Autodesk Fusion 360 part; units mm, degrees
(part 2 of 2)
sketch "Sketch1" plane through (0, 0, 0) normal (1, 0, 0) x (0, 1, 0)
  line L0 (25.4, 0) -> (25.4, -3.175)
  line L1 (12.7, 0) -> (12.7, -3.175)
  line L2 (76.2, 25.4) -> (76.2, 12.7)
  line L3 (0, 0) -> (0, 25.4)
  line L4 (0, 12.7) -> (-3.175, 12.7)
  line L5 (76.2, 12.7) -> (79.375, 12.7)
  line L6 (-3.175, 25.4) -> (0, 25.4)
  line L7 (63.5, -3.175) -> (63.5, 0)
  line L8 (50.8, 0) -> (50.8, -3.175)
  line L9 (79.375, 12.7) -> (79.375, 25.4)
  line L10 (0, -3.175) -> (0, 0)
  line L11 (0, 0) -> (0, 12.7)
  line L12 (25.4, -3.175) -> (38.1, -3.175)
  line L13 (-3.175, 12.7) -> (-3.175, 25.4)
  line L14 (79.375, 25.4) -> (76.2, 25.4)
  line L15 (0, 0) -> (-7.62, 0)
  line L16 (0, 0) -> (-5.715, 0)
  line L17 (-5.715, 0) -> (-5.715, 38.1)
  line L18 (-5.715, 38.1) -> (-5.715, 43.815)
  line L19 (-5.715, 43.815) -> (76.2, 43.815)
  line L20 (76.2, 43.815) -> (81.915, 43.815)
  line L21 (81.915, 43.815) -> (81.915, 0)
  line L22 (81.915, 0) -> (81.915, -5.715)
  line L23 (81.915, -5.715) -> (0, -5.715)
  line L24 (0, -5.715) -> (-5.715, -5.715)
  line L25 (-5.715, -5.715) -> (-5.715, 0)
  line L26 (-5.715, 43.815) -> (12.7, 43.815)
  line L27 (12.7, 43.815) -> (12.7, 40.64)
  line L28 (12.7, 40.64) -> (12.7, 27.94)
  line L29 (81.915, 43.815) -> (63.5, 43.815)
  line L30 (63.5, 43.815) -> (63.5, 27.94)
  line L31 (63.5, 27.94) -> (12.7, 27.94)
  line L32 (12.7, 40.64) -> (63.5, 40.64)
  line L33 (63.5, -3.175) -> (50.8, -3.175)
  line L34 (63.5, 0) -> (50.8, 0)
  line L35 (25.4, -3.175) -> (12.7, -3.175)
  line L36 (12.7, 0) -> (25.4, 0)
  dimension "d2" = 12.7
  dimension "d3" = 3.175
  dimension "d4" = 12.7
  dimension "d6" = 12.7
  dimension "d9" = 12.7
  dimension "d10" = 3.175
  dimension "d12" = 12.7
  dimension "d13" = 3.175
  dimension "d14" = 12.7
  dimension "d16" = 3.175
  dimension "d17" = 12.7
  dimension "d18" = 7.62
  dimension "d21" = 5.715
  dimension "d22" = 5.715
  dimension "d23" = 5.715
  dimension "d24" = 5.715
  dimension "d25" = 3.175
  dimension "d26" = 12.7
  dimension "d27" = 18.415
  constraint coincident L3.start L10.end
  constraint perpendicular L0 L12
  constraint perpendicular L3 L4
  constraint perpendicular L4 L13
  constraint perpendicular L3 L6
  constraint perpendicular L2 L5
  constraint perpendicular L5 L9
  constraint perpendicular L2 L14
  constraint perpendicular L3 L15
  constraint perpendicular L3 L16
  constraint perpendicular L15 L17
  constraint perpendicular L15 L18
  constraint perpendicular L18 L19
  constraint perpendicular L18 L20
  constraint perpendicular L20 L21
  constraint perpendicular L20 L22
  constraint perpendicular L22 L23
  constraint perpendicular L22 L24
  constraint perpendicular L15 L25
  constraint coincident L19 L26.end
  constraint perpendicular L18 L26
  constraint perpendicular L26 L27
  constraint parallel L27 L28
  constraint perpendicular L21 L29
  constraint perpendicular L19 L30
  constraint coincident L30 L32.end
  constraint perpendicular L30 L32
  constraint perpendicular L8 L33
  constraint perpendicular L8 L34
  constraint perpendicular L1 L35
  constraint perpendicular L0 L36
  measures "d2" distance of L1.start L3.start
  measures "d3" distance of L1.start L1.end
  measures "d4" distance of L1.start L0.start
  measures "d6" distance of L0.end L12.end
  measures "d9" distance of L7.end L8.start
  measures "d10" distance of L8.start L8.end
  measures "d12" distance of L3.start L4.start
  measures "d13" distance of L4.end L4.start
  measures "d14" distance of L6.start L4.end
  measures "d16" distance of L5.end L2.end
  measures "d17" distance of L5.end L9.end
  measures "d18" distance of L3.start L15.end
  measures "d21" distance of L3.start L16.end
  measures "d22" distance of L17.end L18.end
  measures "d23" distance of L19.end L20.end
  measures "d24" distance of L21.end L22.end
  measures "d25" distance of L26.end L27.end
  measures "d26" distance of L27.end L28.end
  measures "d27" distance of L20.end L29.end
extrude "Extrude1" add sketch "Sketch1" along normal blind 3.175 contours L17 L18 L19 L20 L21 L22 L23 L24 L25 L26 L27 L28 L29 L30 L31 | L19 L27 L30 L32

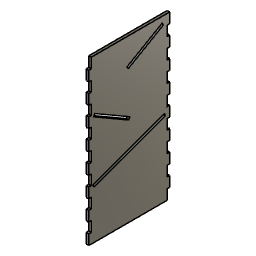
design "Dice Tower (Right Side)"
Autodesk Fusion 360 part; units mm, degrees
sketch "Sketch1" plane through (0, 0, 0) normal (1, 0, 0) x (0, 1, 0)
  line L0 (98.425, 139.7) -> (101.6, 139.7)
  line L1 (0, 101.6) -> (0, 114.3)
  line L2 (0, 127) -> (0, 139.7)
  line L3 (98.425, 114.3) -> (101.6, 114.3)
  line L4 (0, 127) -> (3.175, 127)
  line L5 (101.6, 101.6) -> (101.6, 88.9)
  line L6 (0, 101.6) -> (3.175, 101.6)
  line L7 (98.425, 0) -> (98.425, 203.2)
  line L8 (98.425, 114.3) -> (98.425, 101.6)
  line L9 (98.425, 88.9) -> (101.6, 88.9)
  line L10 (101.6, 0) -> (100.0125, 0)
  line L11 (98.425, 127) -> (101.6, 127)
  line L12 (98.425, 101.6) -> (101.6, 101.6)
  line L13 (98.425, 95.25) -> (98.425, 88.9)
  line L14 (3.175, 0) -> (3.175, 203.2)
  line L15 (101.6, 127) -> (101.6, 114.3)
  line L16 (3.175, 127) -> (3.175, 114.3)
  line L17 (3.175, 88.9) -> (0, 88.9)
  line L18 (98.425, 139.7) -> (98.425, 127)
  line L19 (3.175, 114.3) -> (0, 114.3)
  line L20 (3.175, 12.7) -> (3.175, 0)
  line L21 (3.175, 190.5) -> (3.175, 177.8)
  line L22 (3.175, 177.8) -> (0, 177.8)
  line L23 (101.6, 50.8) -> (101.6, 38.1)
  line L24 (3.175, 50.8) -> (3.175, 38.1)
  line L25 (98.425, 152.4) -> (101.6, 152.4)
  line L26 (98.425, 50.8) -> (101.6, 50.8)
  line L27 (98.425, 152.4) -> (98.425, 139.7)
  line L28 (3.175, 139.7) -> (0, 139.7)
  line L29 (0, 139.7) -> (0, 127)
  line L30 (3.175, 101.6) -> (3.175, 88.9)
  line L31 (98.425, 101.6) -> (98.425, 95.25)
  line L32 (98.425, 203.2) -> (98.425, 190.5)
  line L33 (101.6, 152.4) -> (101.6, 139.7)
  line L34 (101.6, 203.2) -> (101.6, 190.5)
  line L35 (3.175, 203.2) -> (3.175, 190.5)
  line L36 (0, 0) -> (11.0998, 0)
  line L37 (98.425, 177.8) -> (98.425, 165.1)
  line L38 (98.425, 127) -> (98.425, 114.3)
  line L39 (0, 165.1) -> (0, 152.4)
  line L40 (11.0998, 0) -> (6.0198, 0)
  line L41 (98.425, 88.9) -> (98.425, 76.2)
  line L42 (0, 38.1) -> (3.175, 38.1)
  line L43 (98.425, 38.1) -> (98.425, 25.4)
  line L44 (101.6, 177.8) -> (101.6, 165.1)
  line L45 (98.425, 12.7) -> (101.6, 12.7)
  line L46 (0, 177.8) -> (0, 190.5)
  line L47 (98.425, 177.8) -> (101.6, 177.8)
  line L48 (0, 76.2) -> (0, 88.9)
  line L49 (0, 114.3) -> (0, 101.6)
  line L50 (3.175, 190.5) -> (0, 190.5)
  line L51 (98.425, 190.5) -> (101.6, 190.5)
  line L52 (101.6, 0) -> (0, 0)
  line L53 (98.425, 38.1) -> (101.6, 38.1)
  line L54 (90.5002, 0) -> (95.5802, 0)
  line L55 (3.175, 203.2) -> (101.6, 203.2)
  line L56 (98.425, 76.2) -> (101.6, 76.2)
  line L57 (98.425, 165.1) -> (101.6, 165.1)
  line L58 (98.425, 63.5) -> (98.425, 50.8)
  line L59 (98.425, 25.4) -> (101.6, 25.4)
  line L60 (0, 0) -> (0, 12.7)
  line L61 (3.175, 63.5) -> (0, 63.5)
  line L62 (98.425, 63.5) -> (101.6, 63.5)
  line L63 (0, 152.4) -> (0, 165.1)
  line L64 (0, 152.4) -> (3.175, 152.4)
  line L65 (0, 25.4) -> (0, 38.1)
  line L66 (0, 0) -> (12.065, 0)
  line L67 (3.175, 50.8) -> (0, 50.8)
  line L68 (101.6, 203.2) -> (98.425, 203.2)
  line L69 (98.425, 190.5) -> (98.425, 177.8)
  line L70 (101.6, 76.2) -> (101.6, 63.5)
  line L71 (101.6, 0) -> (90.5002, 0)
  line L72 (3.175, 25.4) -> (3.175, 12.7)
  line L73 (98.425, 25.4) -> (98.425, 12.7)
  line L74 (3.175, 38.1) -> (3.175, 25.4)
  line L75 (0, 12.7) -> (3.175, 12.7)
  line L76 (0, 50.8) -> (0, 63.5)
  line L77 (0, 25.4) -> (3.175, 25.4)
  line L78 (3.175, 177.8) -> (3.175, 165.1)
  line L79 (101.6, 0) -> (98.425, 0)
  line L80 (101.6, 0) -> (85.725, 0)
  line L81 (101.6, 25.4) -> (101.6, 12.7)
  line L82 (3.175, 76.2) -> (0, 76.2)
  line L83 (98.425, 165.1) -> (98.425, 152.4)
  line L84 (3.175, 63.5) -> (3.175, 50.8)
  line L85 (3.175, 152.4) -> (3.175, 139.7)
  line L86 (98.425, 76.2) -> (98.425, 63.5)
  line L87 (3.175, 165.1) -> (0, 165.1)
  line L88 (98.425, 50.8) -> (98.425, 38.1)
  line L89 (3.175, 76.2) -> (3.175, 63.5)
  line L90 (0, 0) -> (3.175, 0)
  line L91 (3.175, 88.9) -> (3.175, 76.2)
  line L92 (98.425, 203.2) -> (98.425, 177.8)
  line L93 (3.175, 0) -> (3.175, 59.055)
  line L94 (7.62, 139.7) -> (51.5837, 114.2474)
  line L95 (49.9801, 111.4777) -> (6.0165, 136.9303)
  line L96 (6.0165, 136.9303) -> (7.62, 139.7)
  line L97 (93.7411, 193.04) -> (49.7434, 167.6463)
  line L98 (92.1413, 195.8119) -> (93.7411, 193.04)
  line L99 (48.1436, 170.4182) -> (92.1413, 195.8119)
  line L100 (3.175, 60.2676) -> (4.1957, 60.2676)
  line L101 (4.1957, 60.2676) -> (6.35, 60.2676)
  line L102 (6.35, 60.2676) -> (95.8689, 92.8088)
  line L103 (94.7755, 95.8167) -> (5.2566, 63.2754)
  line L104 (49.9801, 111.4777) -> (50.2, 111.3504)
  line L105 (50.2, 111.3504) -> (51.8035, 114.1201)
  line L106 (51.8035, 114.1201) -> (51.5837, 114.2474)
  line L107 (95.8689, 92.8088) -> (96.1076, 92.8956)
  line L108 (96.1076, 92.8956) -> (95.0142, 95.9034)
  line L109 (95.0142, 95.9034) -> (94.7755, 95.8167)
  line L110 (49.7434, 167.6463) -> (49.5234, 167.5194)
  line L111 (49.5234, 167.5194) -> (47.9236, 170.2912)
  line L112 (47.9236, 170.2912) -> (48.1436, 170.4182)
  line L113 (5.2566, 63.2754) -> (6.35, 60.2676)
  dimension "d9" = 11.0998
  dimension "d10" = 11.0998
  dimension "d14" = 5.08
  dimension "d15" = 5.08
  dimension "d27" = 3.175
  dimension "d28" = 3.175
  dimension "d40" = 3.175
  dimension "d41" = 3.175
  dimension "d42" = 12.7
  dimension "d43" = 12.7
  dimension "d44" = 12.7
  dimension "d45" = 12.7
  dimension "d46" = 12.7
  dimension "d47" = 12.7
  dimension "d48" = 12.7
  dimension "d49" = 12.7
  dimension "d50" = 6.35
  dimension "d51" = 6.35
  dimension "d52" = 12.7
  dimension "d53" = 12.7
  dimension "d54" = 12.7
  dimension "d55" = 12.7
  dimension "d56" = 12.7
  dimension "d57" = 12.7
  dimension "d74" = 59.055
  dimension "d78" = 50.8
  dimension "d79" = 3.2004
  dimension "d80" = 50.8
  dimension "d81" = 50.8
  dimension "d82" = 3.2004
  dimension "d83" = 50.8
  dimension "d84" = 95.25
  dimension "d85" = 3.2004
  dimension "d86" = 95.25
  dimension "d87" = 0.254
  dimension "d88" = 0.254
  dimension "d89" = 3.2004
  dimension "d90" = 0.254
  dimension "d91" = 3.2004
  constraint coincident L36.start L52.end
  constraint vertical L60
  constraint perpendicular L55 L60
  constraint perpendicular L34 L55
  constraint perpendicular L52 L60
  constraint perpendicular L60 L66
  constraint perpendicular L34 L80
  constraint perpendicular L10 L34
  constraint coincident L54.start L52
  constraint perpendicular L36 L60
  constraint perpendicular L50 L60
  constraint perpendicular L21 L50
  constraint coincident L22.end L60
  constraint perpendicular L22 L60
  constraint perpendicular L22 L78
  constraint perpendicular L60 L87
  constraint collinear L46 L60
  constraint perpendicular L39 L87
  constraint perpendicular L39 L64
  constraint parallel L66 L90
  constraint perpendicular L14 L55
  constraint perpendicular L64 L85
  constraint perpendicular L28 L60
  constraint perpendicular L28 L29
  constraint coincident L4.end L14
  constraint perpendicular L4 L14
  constraint perpendicular L4 L16
  constraint perpendicular L16 L19
  constraint perpendicular L19 L49
  constraint midpoint L6.end L14
  constraint perpendicular L6 L14
  constraint perpendicular L6 L30
  constraint parallel L14 L91
  constraint parallel L14 L89
  constraint parallel L14 L84
  constraint parallel L14 L24
  constraint parallel L24 L74
  constraint parallel L14 L72
  constraint perpendicular L17 L60
  constraint coincident L48.start L60
  constraint perpendicular L60 L82
  constraint perpendicular L60 L61
  constraint coincident L67.end L60
  constraint perpendicular L60 L67
  constraint coincident L65.start L60
  constraint collinear L60 L63
  constraint collinear L2 L60
  constraint collinear L1 L60
  constraint collinear L48 L60
  constraint collinear L60 L76
  constraint collinear L60 L65
  constraint perpendicular L34 L68
  constraint perpendicular L34 L79
  constraint perpendicular L32 L55
  constraint perpendicular L34 L51
  constraint perpendicular L51 L69
  constraint coincident L44.start L34
  constraint perpendicular L34 L47
  constraint perpendicular L37 L47
  constraint coincident L44.end L34
  constraint perpendicular L34 L57
  constraint perpendicular L57 L83
  constraint coincident L25.end L34
  constraint perpendicular L25 L34
  constraint perpendicular L25 L27
  constraint coincident L0.end L34
  constraint perpendicular L0 L34
  constraint perpendicular L0 L18
  constraint coincident L11.end L34
  constraint perpendicular L11 L34
  constraint perpendicular L11 L38
  constraint coincident L3.end L34
  constraint perpendicular L3 L34
  constraint perpendicular L3 L8
  constraint perpendicular L12 L34
  constraint perpendicular L12 L31
  constraint parallel L7 L13
  constraint coincident L5.end L34
  constraint perpendicular L9 L34
  constraint perpendicular L9 L41
  constraint coincident L56.end L34
  constraint perpendicular L34 L56
  constraint perpendicular L56 L86
  constraint coincident L62.end L34
  constraint perpendicular L34 L62
  constraint perpendicular L58 L62
  constraint coincident L23.start L34
  constraint perpendicular L26 L34
  constraint perpendicular L26 L88
  constraint coincident L23.end L34
  constraint perpendicular L34 L53
  constraint perpendicular L43 L53
  constraint perpendicular L43 L59
  constraint perpendicular L59 L73
  constraint perpendicular L45 L73
  constraint collinear L34 L44
  constraint coincident L5.start L34
  constraint collinear L33 L44
  constraint collinear L15 L33
  constraint collinear L5 L15
  constraint collinear L5 L70
  constraint collinear L23 L70
  constraint collinear L23 L81
  constraint coincident L84 L93.end
  constraint coincident L84 L100.start
  constraint perpendicular L84 L100
  constraint perpendicular L93 L101
  constraint perpendicular L95 L105
  constraint parallel L102 L107
  constraint perpendicular L107 L108
  constraint parallel L97 L110
  constraint perpendicular L110 L111
  constraint perpendicular L111 L112
  constraint perpendicular L102 L113
  measures "d9" distance of L10.start L54.start
  measures "d10" distance of L36.start L36.end
  measures "d14" distance of L36.end L40.end
  measures "d15" distance of L54.end L54.start
  measures "d27" distance of L39.end L64.end
  measures "d28" distance of L36.start L14.start
  measures "d40" distance of L7.end L34.start
  measures "d41" distance of L7.start L10.start
  measures "d42" distance of L7.end L32.end
  measures "d43" distance of L32.end L37.start
  measures "d44" distance of L37.end L37.start
  measures "d45" distance of L25.start L37.end
  measures "d46" distance of L0.start L25.start
  measures "d47" distance of L0.start L11.start
  measures "d48" distance of L3.start L11.start
  measures "d49" distance of L8.end L3.start
  measures "d50" distance of L8.end L13.start
  measures "d51" distance of L13.start L9.start
  measures "d52" distance of L9.start L41.end
  measures "d53" distance of L41.end L58.start
  measures "d54" distance of L58.start L26.start
  measures "d55" distance of L26.start L43.start
  measures "d56" distance of L43.end L43.start
  measures "d57" distance of L43.end L45.start
  measures "d74" distance of L14.start L93.end
  measures "d78" distance of L94.start L94.end
  measures "d79" distance of L95.start L94.end
  measures "d80" distance of L95.start L95.end
  measures "d81" distance of L97.start L97.end
  measures "d82" distance of L99.start L97.end
  measures "d83" distance of L98.start L99.start
  measures "d84" distance of L101.end L102.end
  measures "d85" distance of L102.end L103.start
  measures "d86" distance of L103.start L103.end
  measures "d87" distance of L95.start L104.end
  measures "d88" distance of L102.end L107.end
  measures "d89" distance of L107.end L108.end
  measures "d90" distance of L97.end L110.end
  measures "d91" distance of L110.end L111.end
extrude "Extrude1" add sketch "Sketch1" along normal blind 3.175
sketch "Sketch2" plane through (0, 0, 0) normal (1, 0, 0) x (0, 1, 0)
equation "d9 = 0.5 in - 0.063 in"

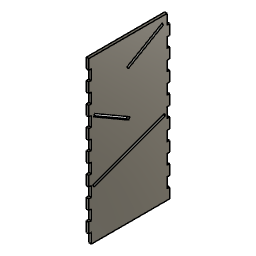
design "Dice Tower (Left Side)"
Autodesk Fusion 360 part; units mm, degrees
sketch "Sketch1" plane through (0, 0, 0) normal (1, 0, 0) x (0, 1, 0)
  line L0 (-98.425, 88.9) -> (-101.6, 88.9)
  line L1 (-98.425, 38.1) -> (-98.425, 25.4)
  line L2 (-98.425, 76.2) -> (-101.6, 76.2)
  line L3 (-101.6, 0) -> (-100.0125, 0)
  line L4 (-98.425, 190.5) -> (-98.425, 177.8)
  line L5 (-101.6, 203.2) -> (-98.425, 203.2)
  line L6 (-98.425, 177.8) -> (-98.425, 165.1)
  line L7 (-98.425, 203.2) -> (-98.425, 177.8)
  line L8 (-3.175, 177.8) -> (0, 177.8)
  line L9 (-98.425, 127) -> (-101.6, 127)
  line L10 (-3.175, 165.1) -> (0, 165.1)
  line L11 (-98.425, 165.1) -> (-98.425, 152.4)
  line L12 (0, 12.7) -> (-3.175, 12.7)
  line L13 (0, 127) -> (-3.175, 127)
  line L14 (-101.6, 76.2) -> (-101.6, 63.5)
  line L15 (-98.425, 63.5) -> (-98.425, 50.8)
  line L16 (-98.425, 114.3) -> (-98.425, 101.6)
  line L17 (-101.6, 101.6) -> (-101.6, 88.9)
  line L18 (-101.6, 0) -> (-98.425, 0)
  line L19 (-98.425, 63.5) -> (-101.6, 63.5)
  line L20 (-101.6, 0) -> (-90.5002, 0)
  line L21 (-3.175, 190.5) -> (-3.175, 177.8)
  line L22 (-3.175, 50.8) -> (0, 50.8)
  line L23 (0, 25.4) -> (-3.175, 25.4)
  line L24 (-3.175, 152.4) -> (-3.175, 139.7)
  line L25 (0, 38.1) -> (-3.175, 38.1)
  line L26 (-101.6, 177.8) -> (-101.6, 165.1)
  line L27 (0, 0) -> (-3.175, 0)
  line L28 (-3.175, 190.5) -> (0, 190.5)
  line L29 (-3.175, 50.8) -> (-3.175, 38.1)
  line L30 (-101.6, 203.2) -> (-101.6, 190.5)
  line L31 (-101.6, 127) -> (-101.6, 114.3)
  line L32 (-98.425, 114.3) -> (-101.6, 114.3)
  line L33 (0, 0) -> (-11.0998, 0)
  line L34 (-98.425, 139.7) -> (-98.425, 127)
  line L35 (-3.175, 177.8) -> (-3.175, 165.1)
  line L36 (-98.425, 165.1) -> (-101.6, 165.1)
  line L37 (-11.0998, 0) -> (-6.0198, 0)
  line L38 (0, 152.4) -> (-3.175, 152.4)
  line L39 (0, 0) -> (-12.065, 0)
  line L40 (-3.175, 76.2) -> (-3.175, 63.5)
  line L41 (-3.175, 139.7) -> (0, 139.7)
  line L42 (-3.175, 12.7) -> (-3.175, 0)
  line L43 (-90.5002, 0) -> (-95.5802, 0)
  line L44 (-98.425, 101.6) -> (-101.6, 101.6)
  line L45 (-3.175, 101.6) -> (-3.175, 88.9)
  line L46 (-3.175, 0) -> (-3.175, 59.055)
  line L47 (-3.175, 88.9) -> (-3.175, 76.2)
  line L48 (-98.425, 177.8) -> (-101.6, 177.8)
  line L49 (-3.175, 38.1) -> (-3.175, 25.4)
  line L50 (-98.425, 152.4) -> (-98.425, 139.7)
  line L51 (-98.425, 203.2) -> (-98.425, 190.5)
  line L52 (-98.425, 139.7) -> (-101.6, 139.7)
  line L53 (-3.175, 63.5) -> (0, 63.5)
  line L54 (-3.175, 203.2) -> (-3.175, 190.5)
  line L55 (-98.425, 127) -> (-98.425, 114.3)
  line L56 (-3.175, 63.5) -> (-3.175, 50.8)
  line L57 (-3.175, 88.9) -> (0, 88.9)
  line L58 (-3.175, 114.3) -> (0, 114.3)
  line L59 (0, 101.6) -> (-3.175, 101.6)
  line L60 (-3.175, 127) -> (-3.175, 114.3)
  line L61 (-98.425, 190.5) -> (-101.6, 190.5)
  line L62 (-98.425, 0) -> (-98.425, 203.2)
  line L63 (-3.175, 76.2) -> (0, 76.2)
  line L64 (-98.425, 152.4) -> (-101.6, 152.4)
  line L65 (-98.425, 25.4) -> (-98.425, 12.7)
  line L66 (-101.6, 152.4) -> (-101.6, 139.7)
  line L67 (-98.425, 38.1) -> (-101.6, 38.1)
  line L68 (-101.6, 0) -> (0, 0)
  line L69 (-98.425, 50.8) -> (-101.6, 50.8)
  line L70 (-101.6, 50.8) -> (-101.6, 38.1)
  line L71 (-98.425, 50.8) -> (-98.425, 38.1)
  line L72 (-101.6, 0) -> (-85.725, 0)
  line L73 (-3.175, 0) -> (-3.175, 203.2)
  line L74 (-98.425, 101.6) -> (-98.425, 95.25)
  line L75 (-98.425, 95.25) -> (-98.425, 88.9)
  line L76 (-3.175, 203.2) -> (-101.6, 203.2)
  line L77 (-98.425, 88.9) -> (-98.425, 76.2)
  line L78 (-3.175, 25.4) -> (-3.175, 12.7)
  line L79 (-98.425, 76.2) -> (-98.425, 63.5)
  line L80 (-101.6, 25.4) -> (-101.6, 12.7)
  line L81 (-98.425, 12.7) -> (-101.6, 12.7)
  line L82 (-98.425, 25.4) -> (-101.6, 25.4)
  line L83 (-6.8245, 95.8167) -> (-96.3434, 63.2754)
  line L84 (-53.6764, 170.2912) -> (-53.4564, 170.4182)
  line L85 (-6.5858, 95.9034) -> (-6.8245, 95.8167)
  line L86 (-51.6199, 111.4777) -> (-51.4, 111.3504)
  line L87 (-7.8589, 193.04) -> (-51.8566, 167.6463)
  line L88 (-95.5835, 136.9303) -> (-93.98, 139.7)
  line L89 (-9.4587, 195.8119) -> (-7.8589, 193.04)
  line L90 (-51.8566, 167.6463) -> (-52.0766, 167.5194)
  line L91 (-5.4924, 92.8956) -> (-6.5858, 95.9034)
  line L92 (-51.6199, 111.4777) -> (-95.5835, 136.9303)
  line L93 (-93.98, 139.7) -> (-50.0163, 114.2474)
  line L94 (-96.3434, 63.2754) -> (-95.25, 60.2676)
  line L95 (-53.4564, 170.4182) -> (-9.4587, 195.8119)
  line L96 (-5.7311, 92.8088) -> (-5.4924, 92.8956)
  line L97 (-51.4, 111.3504) -> (-49.7965, 114.1201)
  line L98 (-95.25, 60.2676) -> (-5.7311, 92.8088)
  line L99 (-49.7965, 114.1201) -> (-50.0163, 114.2474)
  line L100 (-52.0766, 167.5194) -> (-53.6764, 170.2912)
  line L101 (0, 190.5) -> (0, 177.8)
  line L102 (0, 165.1) -> (0, 152.4)
  line L103 (0, 139.7) -> (0, 127)
  line L104 (0, 114.3) -> (0, 101.6)
  line L105 (0, 88.9) -> (0, 76.2)
  line L106 (0, 63.5) -> (0, 50.8)
  line L107 (0, 38.1) -> (0, 25.4)
  line L108 (0, 12.7) -> (0, 0)
  dimension "d92" = 50.8
  dimension "d93" = 3.2004
  dimension "d94" = 50.8
  dimension "d95" = 50.8
  dimension "d96" = 3.2004
  dimension "d97" = 50.8
  dimension "d98" = 95.25
  dimension "d99" = 3.2004
  dimension "d100" = 95.25
  dimension "d101" = 0.254
  dimension "d102" = 0.254
  dimension "d103" = 3.2004
  dimension "d104" = 0.254
  dimension "d105" = 3.2004
  constraint perpendicular L92 L97
  constraint parallel L96 L98
  constraint perpendicular L91 L96
  constraint parallel L87 L90
  constraint perpendicular L90 L100
  constraint perpendicular L84 L100
  constraint perpendicular L94 L98
  constraint perpendicular L8 L101
  constraint perpendicular L38 L102
  constraint perpendicular L13 L103
  constraint perpendicular L59 L104
  constraint perpendicular L63 L105
  constraint perpendicular L22 L106
  constraint parallel L106 L107
  constraint perpendicular L27 L108
  measures "d92" distance of L88.end L93.end
  measures "d93" distance of L93.end L86.start
  measures "d94" distance of L88.start L86.start
  measures "d95" distance of L87.start L87.end
  measures "d96" distance of L84.end L87.end
  measures "d97" distance of L84.end L89.start
  measures "d98" distance of L94.end L96.start
  measures "d99" distance of L96.start L83.start
  measures "d100" distance of L83.end L83.start
  measures "d101" distance of L86.start L86.end
  measures "d102" distance of L96.start L91.start
  measures "d103" distance of L85.start L91.start
  measures "d104" distance of L90.end L87.end
  measures "d105" distance of L84.start L90.end
extrude "Extrude1" add sketch "Sketch1" along normal blind 3.175
sketch "Sketch2" plane through (0, 0, 0) normal (1, 0, 0) x (0, 1, 0)

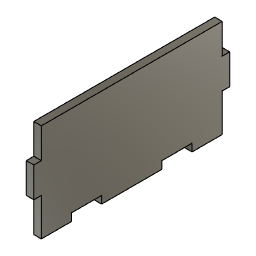
design "Drawer Back (1x)"
Autodesk Fusion 360 part; units mm, degrees
sketch "Sketch1" plane through (0, 0, 0) normal (1, 0, 0) x (0, 1, 0)
  line L0 (0, 0) -> (76.2, 0)
  line L1 (0, 0) -> (12.7, 0)
  line L2 (12.7, 0) -> (12.7, -3.175)
  line L3 (12.7, -3.175) -> (0, -3.175)
  line L4 (0, -3.175) -> (0, 0)
  line L5 (12.7, 0) -> (25.4, 0)
  line L6 (25.4, 0) -> (25.4, -3.175)
  line L7 (25.4, -3.175) -> (38.1, -3.175)
  line L8 (76.2, 0) -> (76.2, -3.175)
  line L9 (76.2, -3.175) -> (63.5, -3.175)
  line L10 (63.5, -3.175) -> (63.5, 0)
  line L11 (63.5, 0) -> (50.8, 0)
  line L12 (50.8, 0) -> (50.8, -3.175)
  line L13 (50.8, -3.175) -> (38.1, -3.175)
  line L14 (0, 0) -> (0, 38.1)
  line L15 (0, 38.1) -> (76.2, 38.1)
  line L16 (76.2, 38.1) -> (76.2, 0)
  line L17 (0, 0) -> (0, 12.7)
  line L18 (0, 12.7) -> (-3.175, 12.7)
  line L19 (-3.175, 12.7) -> (-3.175, 25.4)
  line L20 (-3.175, 25.4) -> (0, 25.4)
  line L21 (76.2, 0) -> (76.2, 12.7)
  line L22 (76.2, 12.7) -> (79.375, 12.7)
  line L23 (79.375, 12.7) -> (79.375, 25.4)
  line L24 (79.375, 25.4) -> (76.2, 25.4)
  dimension "d1" = 76.2
  dimension "d2" = 12.7
  dimension "d3" = 3.175
  dimension "d4" = 12.7
  dimension "d5" = 3.175
  dimension "d6" = 12.7
  dimension "d7" = 3.175
  dimension "d8" = 12.7
  dimension "d9" = 12.7
  dimension "d10" = 3.175
  dimension "d11" = 38.1
  dimension "d12" = 12.7
  dimension "d13" = 3.175
  dimension "d14" = 12.7
  dimension "d15" = 12.7
  dimension "d16" = 3.175
  dimension "d17" = 12.7
  constraint coincident L0.start L1.start
  constraint horizontal L0
  constraint parallel L0 L1
  constraint perpendicular L0 L2
  constraint perpendicular L2 L3
  constraint perpendicular L1 L4
  constraint perpendicular L2 L5
  constraint perpendicular L5 L6
  constraint perpendicular L6 L7
  constraint perpendicular L0 L8
  constraint perpendicular L8 L9
  constraint coincident L0 L10.end
  constraint perpendicular L0 L10
  constraint perpendicular L10 L11
  constraint perpendicular L0 L12
  constraint perpendicular L1 L14
  constraint perpendicular L14 L15
  constraint perpendicular L1 L17
  constraint perpendicular L14 L18
  constraint perpendicular L18 L19
  constraint coincident L14 L20.end
  constraint perpendicular L14 L20
  constraint perpendicular L0 L21
  constraint perpendicular L16 L22
  constraint perpendicular L22 L23
  constraint coincident L16 L24.end
  constraint perpendicular L16 L24
  measures "d1" distance of L0.start L0.end
  measures "d2" distance of L0.start L1.end
  measures "d3" distance of L1.end L2.end
  measures "d4" distance of L1.end L5.end
  measures "d5" distance of L5.end L6.end
  measures "d6" distance of L6.end L7.end
  measures "d7" distance of L0.end L8.end
  measures "d8" distance of L8.end L9.end
  measures "d9" distance of L10.end L11.end
  measures "d10" distance of L11.end L12.end
  measures "d11" distance of L0.start L14.end
  measures "d12" distance of L0.start L17.end
  measures "d13" distance of L17.end L18.end
  measures "d14" distance of L18.end L19.end
  measures "d15" distance of L0.end L21.end
  measures "d16" distance of L21.end L22.end
  measures "d17" distance of L22.end L23.end
extrude "Extrude1" add sketch "Sketch1" along normal blind 3.175
